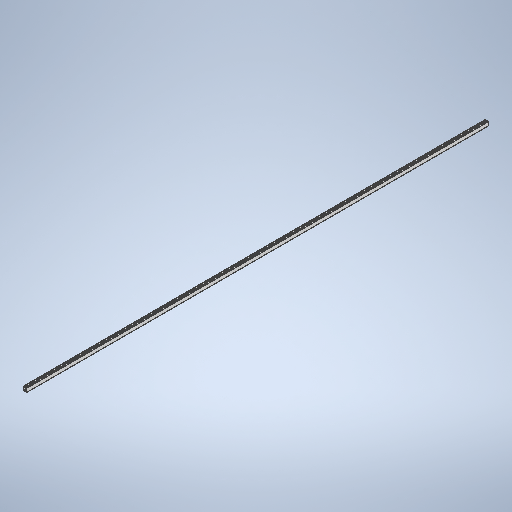
# Autodesk Inventor part: HD - 405 PERFIL ALUMINIO - COLUMNA
Saved by Autodesk Inventor 2025 (Build 290162000, 162)
## iProperties
Created: 2026-01-25
Part Number: HD - 405 PERFIL ALUMINIO - COLUMNA
Material: Generic
Document SubType Name: Modeling
Designer: Frank
Density: 1 g/cm^3
Appearance: Default
Author: Frank
Autodesk Inventor part; units mm, degrees
ref_plane "YZ Plane" through (0, 0, 0) normal (1, 0, 0) x (0, 1, 0)
ref_plane "XZ Plane" through (0, 0, 0) normal (0, 1, 0) x (-1, 0, 0)
ref_plane "XY Plane" through (0, 0, 0) normal (0, 0, 1) x (1, 0, 0)
sketch "Sketch1" plane through (0, 0, 0) normal (0, 0, 1) x (1, 0, 0)
  line L0 (0, 20) -> (0, 0.5)
  line L1 (-0.5, 0) -> (-39.5, 0)
  line L2 (-40, 0.5) -> (-40, 20)
  line L3 (-5.5, 20) -> (-5.5, 3)
  line L4 (-34.5, 3) -> (-34.5, 20)
  line L5 (3.5733, 20) -> (-48.8643, 20) construction
  line L6 (-19.1, 8.9433) -> (-19.1, 8.4104)
  line L7 (-21.1, 8.855) -> (-21.1, 8.3883)
  circle A0 centre (-20, 5.5022) radius 3 construction
  line L8 (-23.3299, 5.7522) -> (-16.6139, 5.7522) construction
  line L9 (-16.6139, 5.7522) -> (-16.6139, 5.2522) construction
  line L10 (-16.6139, 5.2522) -> (-23.3299, 5.2522) construction
  line L11 (-23.3299, 5.2522) -> (-23.3299, 5.7522) construction
  line L12 (-22.7888, 5.7522) -> (-22.9896, 5.7522)
  line L13 (-22.7735, 5.2522) -> (-22.9896, 5.2522)
  arc A1 (-22.9896, 5.7522) -> (-22.9896, 5.2522) centre (-20, 5.5022) ccw
  line L14 (-17.2838, 5.7522) -> (-17.0104, 5.7522)
  line L15 (-17.2265, 5.2522) -> (-17.0104, 5.2522)
  arc A2 (-17.0104, 5.2522) -> (-17.0104, 5.7522) centre (-20, 5.5022) ccw
  arc A3 (-17.2838, 5.7522) -> (-18.8169, 7.9599) centre (-20, 5.5022) ccw
  arc A4 (-21.3576, 7.951) -> (-22.7888, 5.7522) centre (-20, 5.5022) ccw
  arc A5 (-22.7735, 5.2522) -> (-17.2265, 5.2522) centre (-20, 5.5022) ccw
  line L16 (-20.25, 6.2494) -> (-19.75, 6.2494) construction
  line L17 (-19.75, 6.2494) -> (-19.75, 2.1596) construction
  line L18 (-19.75, 2.1596) -> (-20.25, 2.1596) construction
  line L19 (-20.25, 2.1596) -> (-20.25, 6.2494) construction
  line L20 (-20.25, 2.7287) -> (-20.25, 2.5126)
  line L21 (-19.75, 2.5126) -> (-19.75, 2.7287)
  arc A6 (-20.25, 2.5126) -> (-19.75, 2.5126) centre (-20, 4.9859) ccw
  arc A7 (-21.8153, 9.3062) -> (-23.5725, 3.2653) centre (-20, 5.5022) ccw
  arc A8 (-16.4275, 3.2653) -> (-18.4116, 9.4064) centre (-20, 5.5022) ccw
  line L22 (-6, 2.5) -> (-16.0037, 2.5)
  line L23 (-19.75, 2.5) -> (-20.25, 2.5)
  line L24 (-23.9963, 2.5) -> (-34, 2.5)
  circle A9 centre (-20, 5.5022) radius 4.215 construction
  arc A10 (-34.5, 3) -> (-34, 2.5) centre (-34, 3) ccw
  arc A11 (-40, 0.5) -> (-39.5, 0) centre (-39.5, 0.5) ccw
  arc A12 (-23.9963, 2.5) -> (-23.5725, 3.2653) centre (-23.9963, 3) ccw
  arc A13 (-21.1, 8.855) -> (-21.8153, 9.3062) centre (-21.6, 8.855) ccw
  arc A14 (-21.3576, 7.951) -> (-21.1, 8.3883) centre (-21.6, 8.3883) ccw
  arc A15 (-19.1, 8.4104) -> (-18.8169, 7.9599) centre (-18.6, 8.4104) ccw
  arc A16 (-18.4116, 9.4064) -> (-19.1, 8.9433) centre (-18.6, 8.9433) ccw
  arc A17 (-16.4275, 3.2653) -> (-16.0037, 2.5) centre (-16.0037, 3) ccw
  arc A18 (-6, 2.5) -> (-5.5, 3) centre (-6, 3) ccw
  arc A19 (-0.5, 0) -> (0, 0.5) centre (-0.5, 0.5) ccw
  line L25 (0, 20) -> (0, 39.5)
  line L26 (-0.5, 40) -> (-39.5, 40)
  line L27 (-40, 39.5) -> (-40, 20)
  line L28 (-5.5, 20) -> (-5.5, 37)
  line L29 (-34.5, 37) -> (-34.5, 20)
  line L30 (-19.1, 31.0567) -> (-19.1, 31.5896)
  line L31 (-21.1, 31.145) -> (-21.1, 31.6117)
  circle A20 centre (-20, 34.4978) radius 3 construction
  line L32 (-23.3299, 34.2478) -> (-16.6139, 34.2478) construction
  line L33 (-16.6139, 34.2478) -> (-16.6139, 34.7478) construction
  line L34 (-16.6139, 34.7478) -> (-23.3299, 34.7478) construction
  line L35 (-23.3299, 34.7478) -> (-23.3299, 34.2478) construction
  line L36 (-22.7888, 34.2478) -> (-22.9896, 34.2478)
  line L37 (-22.7735, 34.7478) -> (-22.9896, 34.7478)
  arc A21 (-22.9896, 34.7478) -> (-22.9896, 34.2478) centre (-20, 34.4978) ccw
  line L38 (-17.2838, 34.2478) -> (-17.0104, 34.2478)
  line L39 (-17.2265, 34.7478) -> (-17.0104, 34.7478)
  arc A22 (-17.0104, 34.2478) -> (-17.0104, 34.7478) centre (-20, 34.4978) ccw
  arc A23 (-18.8169, 32.0401) -> (-17.2838, 34.2478) centre (-20, 34.4978) ccw
  arc A24 (-22.7888, 34.2478) -> (-21.3576, 32.049) centre (-20, 34.4978) ccw
  arc A25 (-17.2265, 34.7478) -> (-22.7735, 34.7478) centre (-20, 34.4978) ccw
  line L40 (-20.25, 33.7506) -> (-19.75, 33.7506) construction
  line L41 (-19.75, 33.7506) -> (-19.75, 37.8404) construction
  line L42 (-19.75, 37.8404) -> (-20.25, 37.8404) construction
  line L43 (-20.25, 37.8404) -> (-20.25, 33.7506) construction
  line L44 (-20.25, 37.2713) -> (-20.25, 37.4874)
  line L45 (-19.75, 37.4874) -> (-19.75, 37.2713)
  arc A26 (-19.75, 37.4874) -> (-20.25, 37.4874) centre (-20, 35.0141) ccw
  arc A27 (-23.5725, 36.7347) -> (-21.8153, 30.6938) centre (-20, 34.4978) ccw
  arc A28 (-18.4116, 30.5936) -> (-16.4275, 36.7347) centre (-20, 34.4978) ccw
  line L46 (-6, 37.5) -> (-16.0037, 37.5)
  line L47 (-19.75, 37.5) -> (-20.25, 37.5)
  line L48 (-23.9963, 37.5) -> (-34, 37.5)
  circle A29 centre (-20, 34.4978) radius 4.215 construction
  arc A30 (-34, 37.5) -> (-34.5, 37) centre (-34, 37) ccw
  arc A31 (-39.5, 40) -> (-40, 39.5) centre (-39.5, 39.5) ccw
  arc A32 (-23.5725, 36.7347) -> (-23.9963, 37.5) centre (-23.9963, 37) ccw
  arc A33 (-21.8153, 30.6938) -> (-21.1, 31.145) centre (-21.6, 31.145) ccw
  arc A34 (-21.1, 31.6117) -> (-21.3576, 32.049) centre (-21.6, 31.6117) ccw
  arc A35 (-18.8169, 32.0401) -> (-19.1, 31.5896) centre (-18.6, 31.5896) ccw
  arc A36 (-19.1, 31.0567) -> (-18.4116, 30.5936) centre (-18.6, 31.0567) ccw
  arc A37 (-16.0037, 37.5) -> (-16.4275, 36.7347) centre (-16.0037, 37) ccw
  arc A38 (-5.5, 37) -> (-6, 37.5) centre (-6, 37) ccw
  arc A39 (0, 39.5) -> (-0.5, 40) centre (-0.5, 39.5) ccw
  point P0 (0, 0)
  point P1 (0, 0)
  point P2 (-40, 0)
  point P3 (-19.1, 9.62)
  point P4 (-19.1, 8.077)
  point P5 (-21.1, 9.5711)
  point P6 (-21.1, 8.077)
  point P7 (-22.9586, 2.5)
  point P8 (-17.0414, 2.5)
  point P9 (-17.1471, 5.7522)
  point P10 (-17.1185, 5.2522)
  point P11 (0, 40)
  point P12 (-40, 40)
  point P13 (-19.1, 30.38)
  point P14 (-19.1, 31.923)
  point P15 (-21.1, 30.4289)
  point P16 (-21.1, 31.923)
  point P17 (-22.9586, 37.5)
  point P18 (-17.0414, 37.5)
  point P19 (-17.1471, 34.2478)
  point P20 (-17.1185, 34.7478)
  dimension "d2" = 5.5
  dimension "d3" = 5.5
  dimension "d5" = 40
  dimension "d6" = 20
  dimension "d12" = 6
  dimension "d14" = 0.25
  dimension "d16" = 0.25
  dimension "d18" = 20
  dimension "d19" = 8.43
  dimension "d20" = 0.5
  dimension "d21" = 2
  dimension "d23" = 0.5
  dimension "d24" = 2.5
  constraints: 100 point on circle, 98 end point, 69 symmetric about line, 52 point on line, 40 centre point, 24 tangent, 11 equal radius, 7 coincident, 6 parallel, 3 perpendicular, 2 horizontal, 2 midpoint, 2 vertical, 20 other
  measures "d2" distance between parallel lines of L0 L3
  measures "d3" distance between parallel lines of L2 L4
  measures "d5" distance of point (0, 0) point (-40, 0)
  measures "d6" distance between parallel lines of L1 L5
  measures "d12" diameter of A0
  measures "d14" distance from line of A1.centre L19
  measures "d16" distance from line of A3.centre L17
  measures "d18" distance from line of L0 A3.centre
  measures "d19" diameter of A9
  measures "d20" vertical distance of point (-17.147, 5.752) point (-17.118, 5.252)
  measures "d21" distance between parallel lines of L6 L7
  measures "d23" radius of A10
  measures "d24" distance between parallel lines of L1 L22
extrude "Extrusion1" add sketch "Sketch1" against normal blind 5000
body "Solid1"
